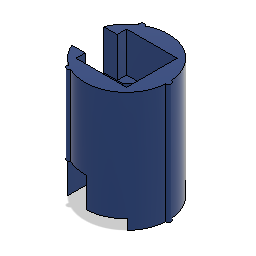
Switch_spacer_2023.04.09 (Autodesk Fusion 360 design; units mm, degrees)
Autodesk Fusion 360 part; units mm, degrees
sketch "Sketch1" plane through (0, 0, 0) normal (0, 1, 0) x (1, 0, 0) in component "SwitchSpacer"
  arc A0 (-5.8311, -8.732) -> (-5.8573, 8.7145) centre (0, 0) cw
  arc A1 (-4.6183, -9.4298) -> (-5.8311, -8.732) centre (-5.2363, -9.1011) cw
  line L0 (-20, 3.982) -> (0, 3.982)
  arc A2 (10.4756, 0.7154) -> (10.4777, -0.6839) centre (10.5, 0.0158) cw
  arc A3 (-4.6466, 9.4159) -> (10.4756, 0.7154) centre (0, 0) cw
  arc A4 (10.4777, -0.6839) -> (-4.6183, -9.4298) centre (0, 0) cw
  arc A5 (-5.8573, 8.7145) -> (-4.6466, 9.4159) centre (-5.2637, 9.0854) cw
  line L1 (-20, -4.0237) -> (-20, 3.982)
  line L2 (0, 3.982) -> (0, -4.0237)
  line L3 (0, -4.0237) -> (-20, -4.0237)
  circle A6 centre (0, 0) radius 6.35
  line L4 (7.5, 12) -> (-7.5, 12)
  line L5 (-7.5, 12) -> (-7.5, -12)
  line L6 (-7.5, -12) -> (7.5, -12)
  line L7 (7.5, -12) -> (7.5, 12)
  line L8 (7.5, 12) -> (-7.5, -12) construction
  line L9 (-7.5, 12) -> (7.5, -12) construction
  line L10 (0.5, -12) -> (0.5, 12)
  line L11 (2, -12) -> (2, 12)
  point P0 (0.5, -12)
  point P1 (0, -12)
  point P2 (2, -12)
  dimension "d39" = 12.7
  dimension "d40" = 15
  dimension "d41" = 24
  dimension "d42" = 0.5
  dimension "d51" = 1.5
  constraint concentric A0 A6
  constraint horizontal L4
  constraint perpendicular L4 L5
  constraint parallel L4 L6
  constraint parallel L5 L7
  constraint coincident L8 A0.centre
  constraint coincident L9 A0.centre
  constraint coincident A0.centre A3.centre
  constraint coincident L6 P0
  constraint midpoint L6 P1
  constraint coincident P0 L10.start
  constraint coincident L4 L10.end
  constraint perpendicular L4 L10
  constraint coincident L6 P2
  constraint coincident P2 L11.start
  constraint coincident L4 L11.end
  constraint perpendicular L4 L11
  measures "d39" diameter of A6
  measures "d40" distance of L5.end L6.end
  measures "d41" distance of L4.end L5.end
  measures "d42" distance of P0 P1
  measures "d51" distance of P0 P2
extrude "Extrude8" add sketch "Sketch1" along normal blind 10 contours A0 A1 A4 L3 A6 L5 L10 | A0 L3 L5 | A4 A6 L10 L11 | A0 L0 L5 | A0 L0 A3 A5 A6 L5 L10 | A3 A4 A6 L7 L11 | A6 L10 L11 | A2 A3 A4 L7 | A6 L11 | A3 A6 L10 L11 in component "SwitchSpacer"
sketch "Sketch2" plane through (0, 10, 0) normal (0, 1, 0) x (-1, 0, 0) in component "SwitchSpacer"
  circle A0 centre (0, 0) radius 4
  line L0 (6.35, 6.35) -> (-6.35, 6.35)
  line L1 (-6.35, 6.35) -> (-6.35, -6.35)
  line L2 (-6.35, -6.35) -> (6.35, -6.35)
  line L3 (6.35, -6.35) -> (6.35, 6.35)
  line L4 (6.35, 6.35) -> (-6.35, -6.35) construction
  line L5 (-6.35, 6.35) -> (6.35, -6.35) construction
  line L6 (6.35, 6.35) -> (19.35, 6.35)
  line L7 (19.35, 6.35) -> (19.35, -6.35)
  line L8 (19.35, -6.35) -> (6.35, -6.35)
  line L9 (6.35, -6.35) -> (6.35, 6.35)
  circle A1 centre (0, 0) radius 6.35
  line L10 (12.5, -3.5) -> (-12.5, -3.5)
  line L11 (-12.5, -3.5) -> (-12.5, 3.5)
  line L12 (-12.5, 3.5) -> (12.5, 3.5)
  line L13 (12.5, 3.5) -> (12.5, -3.5)
  line L14 (12.5, -3.5) -> (-12.5, 3.5) construction
  line L15 (-12.5, -3.5) -> (12.5, 3.5) construction
  arc A2 (9.6985, 4.0237) -> (5.8311, 8.732) centre (0, 0) ccw
  arc A3 (5.8311, 8.732) -> (4.6183, 9.4298) centre (5.2363, 9.1011) ccw
  arc A4 (4.6183, 9.4298) -> (-10.4777, 0.6839) centre (0, 0) ccw
  arc A5 (-10.4777, 0.6839) -> (-10.4756, -0.7154) centre (-10.5, -0.0158) ccw
  arc A6 (-10.4756, -0.7154) -> (4.6466, -9.4159) centre (0, 0) ccw
  arc A7 (4.6466, -9.4159) -> (5.8573, -8.7145) centre (5.2637, -9.0854) ccw
  arc A8 (-0.5, -6.3303) -> (4.9463, -3.982) centre (0, 0) ccw
  line L16 (-0.5, -6.3303) -> (-0.5, 6.3303)
  line L17 (9.7156, -3.982) -> (4.9463, -3.982)
  arc A9 (4.9125, 4.0237) -> (-0.5, 6.3303) centre (0, 0) ccw
  line L18 (4.9125, 4.0237) -> (9.6985, 4.0237)
  arc A10 (5.8573, -8.7145) -> (9.7156, -3.982) centre (0, 0) ccw
  dimension "d18" = 12.7
  dimension "d19" = 12.7
  dimension "d20" = 13
  dimension "d21" = 12.7
  dimension "d22" = 12.7
  dimension "d27" = 25
  dimension "d28" = 7
  constraint horizontal L0
  constraint perpendicular L0 L1
  constraint parallel L0 L2
  constraint parallel L1 L3
  constraint coincident L4 A0.centre
  constraint coincident L5 A0.centre
  constraint coincident A0.centre A1.centre
  constraint horizontal L6
  constraint vertical L7
  constraint horizontal L8
  constraint vertical L9
  constraint horizontal L10
  constraint perpendicular L10 L11
  constraint parallel L10 L12
  constraint parallel L11 L13
  constraint coincident L14 A0.centre
  constraint coincident L15 A0.centre
  measures "d18" distance of L1.end L2.end
  measures "d19" distance of L0.end L1.end
  measures "d20" distance of L0.start L6.end
  measures "d21" distance of L0.start L2.end
  measures "d22" diameter of A1
  measures "d27" distance of L11.end L12.end
  measures "d28" distance of L10.end L11.end
extrude "Extrude10" add sketch "Sketch2" along normal blind 10 contours L0 L1 L6 L12 A2 A3 A4 | L3 L6 L9 A2 L18 | L1 L2 L8 L10 A6 A7 A10 | L3 L8 L9 L17 A10 | L1 L10 L12 A4 A5 A6 in component "SwitchSpacer"
extrude "Extrude12" add sketch "Sketch1" along normal blind 6.5 contours A0 L0 L3 L5 | L0 L3 A6 L5 in component "SwitchSpacer"
extrude "Extrude13" add sketch "Sketch1" against normal blind 10 contours A0 L3 L5 | A0 L0 L3 L5 | A0 L0 L5 | A2 A3 A4 L7 in component "SwitchSpacer"
extrude "Extrude14" add sketch "Sketch1" against normal blind 7.5 contours A4 A6 L10 L11 | A3 A4 A6 L7 L11 | A6 L10 L11 | A6 L11 | A3 A6 L10 L11 in component "SwitchSpacer"
fillet "Fillet1" radius 3.5 2 edges at (-7.331, 6.5, -3.982) (-7.3055, 6.5, 4.0237) in component "SwitchSpacer"
sketch "Sketch3" plane through (0, -7.5, 0) normal (0, -1, 0) x (1, 0, 0) in component "SwitchSpacer"
  line L0 (7.5, -7.3485) -> (7.5, 7.3485)
  arc A0 (7.5, 7.3485) -> (0.5, 10.4881) centre (0, 0) ccw
  line L1 (0.5, 10.4881) -> (0.5, -10.4881)
  arc A1 (0.5, -10.4881) -> (7.5, -7.3485) centre (0, 0) ccw
  circle A2 centre (0, 0) radius 8.5
  line L2 (1.9353, 11.9343) -> (1.9353, -13.1678)
  point P0 (1.9353, 11.9343)
  dimension "d52" = 17
  dimension "d53" = 1.9353
  constraint coincident A0.centre A1.centre
  constraint coincident P0 L2.start
  constraint vertical L2
  measures "d52" diameter of A2
  measures "d53" horizontal distance of A0.centre P0
extrude "Extrude15" cut sketch "Sketch3" against normal blind 14 contours L0 A2 L2 in component "SwitchSpacer"
extrude "Extrude16" add sketch "Sketch3" against normal blind 2 contours L0 A2 L2 in component "SwitchSpacer"
hole "Hole2" at (3.5, 10, 0.35) direction (0, -1, 0) diameter 4 depth 5 tip angle 118 in component "SwitchSpacer"
component "SwitchSpacer" placed x (1, 0, 0) y (0, 1, 0) z (0, 0, 1) at (0, 0, 0)
